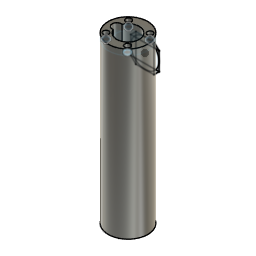
wand hilt 2 (Autodesk Fusion 360 design; units mm, degrees)
part number: 2025-05-15-15-05-41-209
Autodesk Fusion 360 part; units mm, degrees
sketch "Sketch1" plane through (0, 0, 0) normal (0, 0, 1) x (1, 0, 0)
  circle A0 centre (0, 0) radius 17.5
  line L0 (-10, 13) -> (10, 13)
  line L1 (10, 13) -> (10, -13)
  line L2 (10, -13) -> (-10, -13)
  line L3 (-10, -13) -> (-10, 13)
  dimension "d1" = 35
  dimension "d2" = 20
  dimension "d3" = 26
  dimension "d4" = 13
  dimension "d5" = 10
  constraint coincident A0.centre origin
  constraint horizontal L0
  constraint vertical L1
  constraint horizontal L2
  constraint vertical L3
  measures "d1" diameter of A0
  measures "d2" distance of L0.start L0.end
  measures "d3" distance of L0.start L2.end
  measures "d4" distance of A0.centre L0
  measures "d5" distance of A0.centre L1
  measures "d59" distance of A0.centre
extrude "Extrude1" add sketch "Sketch1" along normal blind 65
sketch "Sketch2" plane through (0, 0, 65) normal (0, 0, 1) x (-1, 0, 0)
  line L0 (-10, 13) -> (10, 13)
  line L1 (10, 13) -> (10, -13)
  line L2 (10, -13) -> (-10, -13)
  line L3 (-10, -13) -> (-10, 13)
  circle A0 centre (0, 0) radius 17.5
  circle A1 centre (0, 0) radius 17.5
  constraint concentric A0 A1
extrude "Extrude2" add sketch "Sketch2" along normal blind 2 contours L0 L1 L2 L3 | A0 A1
sketch "Sketch3" plane through (0, 0, 67) normal (0, 0, 1) x (-1, 0, 0)
  circle A0 centre (0, 0) radius 17.5
  circle A1 centre (0, 0) radius 10
  circle A2 centre (9.973, -0.7342) radius 4
  circle A3 centre (-10.4741, -0.0703) radius 3
  dimension "d11" = 20
  dimension "d34" = 8
  dimension "d35" = 6
  constraint coincident A0.centre A1.centre
  measures "d11" diameter of A1
  measures "d34" diameter of A2
  measures "d35" diameter of A3
extrude "Extrude3" add sketch "Sketch3" along normal blind 74 contours A0 | A1 A2 | A1 A3 picked at (11.3007, -0.6406) picked at (-10.9113, 1.0336)
fillet "Fillet1" radius 3 1 edges at (9.3233, 3.6162, 67)
form "Form1" [no effect]
sketch "Sketch4" plane through (0, 0, 0) normal (0, 0, 1) x (1, 0, 0)
  circle A0 centre (-13, 0) radius 2
  circle A1 centre (0, 0) radius 17.5
  circle A2 centre (13, 0) radius 2
  dimension "d16" = 4
  dimension "d17" = 13
  dimension "d18" = 4
  dimension "d19" = 13
  measures "d16" diameter of A0
  measures "d17" distance of A0.centre A1.centre
  measures "d18" diameter of A2
  measures "d19" distance of A2.centre A1.centre
extrude "Extrude4" cut sketch "Sketch4" along normal blind 5 contours A0 | A2
sketch "Sketch5" plane through (0, 0, 141) normal (0, 0, 1) x (-1, 0, 0)
  circle A0 centre (0, 0) radius 10
  circle A1 centre (0, 0) radius 17.5
  circle A2 centre (-9.5039, 10) radius 2.5
  circle A3 centre (10, 9.5039) radius 2.5
  circle A4 centre (9.5039, -10) radius 2.5
  circle A5 centre (-10, -9.5039) radius 2.5
  point P0 (-10, -9.5039)
  point P1 (9.5039, -10)
  point P2 (10, 9.5039)
  dimension "d22" = 5
  dimension "d24" = 10
  dimension "d26" = 360
  dimension "d27" = 5
  dimension "d28" = 5
  dimension "d29" = 5
  constraint coincident P2 A3.centre
  constraint coincident P1 A4.centre
  constraint coincident P0 A5.centre
  measures "d22" diameter of A2
  measures "d24" vertical distance of A0.centre A2.centre
  measures "d27" diameter of A3
  measures "d28" diameter of A4
  measures "d29" diameter of A5
extrude "Extrude5" add sketch "Sketch5" along normal blind 4 contours A2 | A3 | A4 | A5
extrude "Extrude6" cut 4 faces at (-9.0915, -9.8035, 145) (-8.5953, 9.7003, 145) (11.044, 9.7309, 145) (10.9023, -9.8451, 145) along direction (0, 0, -1) blind 5
extrude "Extrude7" cut sketch "Sketch3" along normal blind 76 contours A1 A2 picked at (11.3007, -0.6406)
extrude "Extrude8" cut sketch "Sketch3" against normal blind 17 contours A1 A2 | A1 A2
delete_face "DeleteFace1" 1 faces at (-3.1845, -6.8651, 67.0542)
fillet "Fillet2" radius 0.5 1 edges at (9.973, -0.7342, 67)
fillet "Fillet4" radius 3.5 1 edges at (-13.973, 0.7342, 50)
sketch "Sketch6" plane through (0, 0, 0) normal (0, 1, 0) x (1, 0, 0)
ref_plane "WorkPlane1" through (0, 17.5, 0) normal (0, 1, 0) x (0, 0, 1)
sketch "Sketch7" plane through (0, 17.5, 0) normal (0, 1, 0) x (1, 0, 0)
  circle A0 centre (0, -123) radius 6.15
  circle A1 centre (0, -123) radius 8.725
  dimension "d47" = 17.45
  dimension "d48" = 12.3
  constraint concentric A0 A1
  measures "d47" diameter of A1
  measures "d48" diameter of A0
extrude "Extrude9" cut sketch "Sketch7" against normal blind 13 contours A0
extrude "Extrude10" cut sketch "Sketch7" against normal blind 2.5
sketch "Sketch8" plane through (0, 0, 141) normal (0, 0, 1) x (-1, 0, 0)
  circle A0 centre (0, 0) radius 17.5
  arc A1 (8.8874, -4.5841) -> (9.4629, 3.2331) centre (9.973, -0.7342) ccw
  arc A2 (9.4629, 3.2331) -> (8.8874, -4.5841) centre (0, 0) ccw
  circle A3 centre (10, 9.5039) radius 2.5
  circle A4 centre (9.5039, -10) radius 2.5
  circle A5 centre (-9.5039, 10) radius 2.5
  circle A6 centre (-10, -9.5039) radius 2.5
  circle A7 centre (0, 0) radius 10
  constraint concentric A0 A7
ref_plane "WorkPlane2" through (-0.1339, 0.4405, 134) normal (0, 0, 1) x (-1, 0, 0)
sketch "Sketch9" plane through (0, 0, 134) normal (0, 0, 1) x (1, 0, 0)
  circle A0 centre (0, -6.5) radius 10
  dimension "d55" = 20
  dimension "d59" = 6.5
  measures "d55" diameter of A0
  measures "d59" distance of origin A0.centre
extrude "Extrude11" cut sketch "Sketch9" against normal blind 64
sketch "Sketch10" plane through (0, 0, 134) normal (0, 0, 1) x (1, 0, 0)
  circle A0 centre (-8.5557, -8.8318) radius 4
  circle A1 centre (-9.9246, -6.6871) radius 4
  dimension "d60" = 8
  dimension "d63" = 8
  measures "d60" diameter of A0
  measures "d63" diameter of A1
extrude "Extrude12" cut sketch "Sketch10" against normal blind 100 contours A0 A1 | A0 A1 picked at (-6.6652, -10.2386) picked at (-8.609, -8.4294)
extrude "Extrude13" cut sketch "Sketch10" against normal blind 100 contours A0 A1 | A0 A1 picked at (-8.609, -8.4294) picked at (-11.1603, -4.7512)
fillet "Fillet5" radius 209.5 1 edges at (-12.4368, -9.7998, 84)
sketch "Sketch11" plane through (0, 0, 70) normal (0, 0, 1) x (-1, 0, 0)
  arc A0 (7.7986, 12.7595) -> (4.5563, 8.9017) centre (8.5557, 8.8318) ccw
  arc A1 (7.7986, 12.7595) -> (-9.4571, 3.25) centre (0, 6.5) ccw
  circle A2 centre (10, -0.5) radius 4
  circle A3 centre (-0.3117, 0) radius 10
  arc A4 (4.5563, 8.9017) -> (-9.4571, 3.25) centre (0, 0) ccw
  dimension "d70" = 8
  dimension "d71" = 20
  measures "d70" diameter of A2
  measures "d71" diameter of A3
delete_face "DeleteFace2" 1 faces at (-10.2742, -2.4924, 51.3231)
delete_face "DeleteFace3" 1 faces at (-10.408, 4.7105, 85.3333)
sketch "Sketch12" plane through (0, 0, 141) normal (0, 0, 1) x (-1, 0, 0)
  circle A0 centre (-9.5039, 10) radius 2.5
  circle A1 centre (-10, -9.5039) radius 2.5
  circle A2 centre (10, 9.5039) radius 2.5
  circle A3 centre (0, 0) radius 17.5
  circle A4 centre (9.5039, -10) radius 2.5
  circle A5 centre (0, 0) radius 10
  circle A6 centre (10, 0) radius 4
  dimension "d72" = 8
  constraint coincident A5 A6.centre
  measures "d72" diameter of A6
extrude "Extrude14" cut sketch "Sketch12" against normal blind 46 contours A5 A6 picked at (11.1746, -1.0177)
fillet "Fillet7" radius 3.5 1 edges at (-13.7064, 1.5042, 95)
extrude "Extrude15" add 1 faces at (-4.698, 12.6936, 141) along direction (0, 0, 1) blind 5
extrude "Extrude16" cut sketch "Sketch9" along normal blind 5
extrude "Extrude17" cut sketch "Sketch10" along normal blind 5
fillet "Fillet8" radius 88.75 1 edges at (-12.4368, -9.7998, 136.5)
sketch "Sketch13" plane through (0, 0, 0) normal (0, 0, 1) x (1, 0, 0)
ref_plane "WorkPlane3" through (0, 0, 100) normal (0, 0, 1) x (1, 0, 0)
sketch "Sketch14" plane through (0, 0, 100) normal (0, 0, 1) x (1, 0, 0)
  circle A0 centre (0, 10) radius 4
  dimension "d86" = 8
  measures "d86" diameter of A0
extrude "Extrude18" cut sketch "Sketch14" against normal blind 55
fillet "Fillet9" radius 1.75 1 edges at (0, 14, 45)
extrude "Extrude19" cut sketch "Sketch14" along normal blind 18
extrude "Extrude20" cut sketch "Sketch11" against normal blind 3 contours A0 A1 A3 A4
delete_face "DeleteFace4" 1 faces at (9.0742, 3.7828, 67.1254)
sketch "Sketch15" plane through (0, 0, 0) normal (0, 0, -1) x (1, 0, 0)
  circle A0 centre (13, 0) radius 2
  circle A1 centre (-13, 0) radius 2
  line L0 (-10, 13) -> (10, 13)
  line L1 (10, 13) -> (10, -13)
  line L2 (10, -13) -> (-10, -13)
  line L3 (-10, -13) -> (-10, 13)
  circle A2 centre (0, 0) radius 17.5
  line L4 (10, -11) -> (12, -11)
  line L5 (12, -11) -> (12, -7)
  line L6 (10, -7) -> (10, -11)
  line L7 (12, 6) -> (12, 11)
  line L8 (10, 11) -> (10, 6)
  line L9 (12, 11) -> (10, 11)
  line L10 (-10, -11.7544) -> (-10, -6)
  line L11 (-12, -6) -> (-12, -11)
  line L12 (10, 11) -> (12, 11)
  line L13 (12, 11) -> (12, 5)
  line L14 (12, 5) -> (10, 5)
  line L15 (10, 5) -> (10, 11)
  line L16 (-12.1346, 12.045) -> (-9.6346, 12.045)
  line L17 (-9.6346, 12.045) -> (-9.6347, 5.045)
  line L18 (-9.6347, 5.045) -> (-11.9882, 5.045)
  line L19 (-11.9882, 5.045) -> (-12.1346, 12.045)
  line L20 (-10, -11.7544) -> (-12, -11.7544)
  line L21 (-12, -11.7544) -> (-12, -5)
  line L22 (-12, -5) -> (-10, -5)
  line L23 (-10, -5) -> (-10, -11.7544)
  line L24 (10, -11) -> (12, -11)
  line L25 (12, -11) -> (12, -5)
  line L26 (12, -5) -> (10, -5)
  line L27 (10, -5) -> (10, -11)
  dimension "d98" = 6
  dimension "d101" = 7
  dimension "d102" = 7
  dimension "d103" = 2.5
  constraint horizontal L4
  constraint vertical L5
  constraint vertical L6
  constraint coincident L1 L4.start
  constraint vertical L7
  constraint vertical L8
  constraint horizontal L9
  constraint vertical L10
  constraint vertical L11
  constraint horizontal L12
  constraint horizontal L14
  constraint horizontal L18
  constraint horizontal L22
  constraint horizontal L24
  constraint horizontal L26
  measures "d98" distance of L4.start L26.end
  measures "d101" vertical distance of L16.start L18.end
  measures "d102" distance of L16.end L17.end
  measures "d103" distance of L16.start L16.end
extrude "Extrude21" cut sketch "Sketch15" against normal blind 65 contours L3 L16 L18 L19 | L1 L7 L8 L9 L12 L13 L14 L15 | L3 L10 L11 L20 L21 L22 L23 | L1 L4 L5 L6 L24 L25 L26 L27
sketch "Sketch16" plane through (0, 0, 0) normal (0, 0, 1) x (1, 0, 0)
sketch "Sketch17" plane through (0, 15, 0) normal (0, 1, 0) x (-1, 0, 0)
  circle A0 centre (0, 123) radius 6.15
  circle A1 centre (0, 123) radius 8.725
  circle A2 centre (0, 123) radius 12.5
  line L0 (-8, 135.5) -> (8, 135.5)
  line L1 (8, 135.5) -> (8, 110.5)
  line L2 (8, 110.5) -> (-8, 110.5)
  line L3 (-8, 110.5) -> (-8, 135.5)
  line L4 (-12.5, 131) -> (12.5, 131)
  line L5 (12.5, 131) -> (12.5, 115)
  line L6 (12.5, 115) -> (-12.5, 115)
  line L7 (-12.5, 115) -> (-12.5, 131)
  line L8 (-12.5, 131) -> (-8, 135.5)
  line L9 (8, 135.5) -> (12.5, 131)
  line L10 (12.5, 115) -> (8, 110.5)
  line L11 (-8, 110.5) -> (-12.5, 115)
  dimension "d104" = 25
  dimension "d105" = 16
  dimension "d106" = 25
  dimension "d107" = 25
  dimension "d108" = 16
  dimension "d109" = 12.5
  dimension "d110" = 12.5
  dimension "d111" = 8
  dimension "d112" = 8
  constraint horizontal L0
  constraint vertical L1
  constraint horizontal L2
  constraint vertical L3
  constraint horizontal L4
  constraint vertical L5
  constraint horizontal L6
  constraint vertical L7
  constraint coincident A0.centre A1.centre
  measures "d104" diameter of A2
  measures "d105" distance of L0.start L0.end
  measures "d106" distance of L0.start L2.end
  measures "d107" distance of L4.start L4.end
  measures "d108" distance of L4.start L6.end
  measures "d109" distance of A0.centre L7
  measures "d110" distance of A0.centre L0
  measures "d111" distance of A0.centre L4
  measures "d112" distance of A0.centre L3
